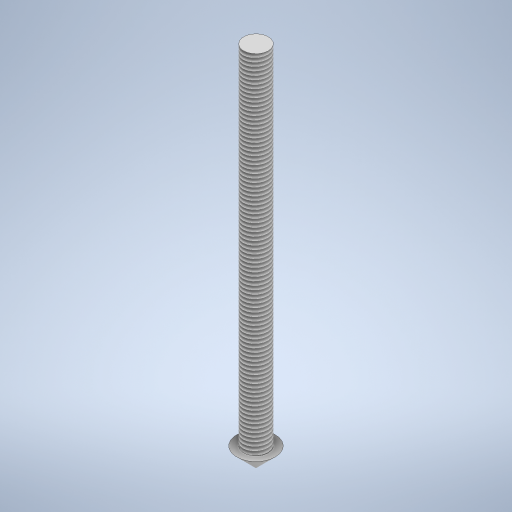
# Autodesk Inventor part: Digging Tool
Saved by Autodesk Inventor 2024 (Build 280153000, 153)
## iProperties
Created: 2024-02-05
Part Number: Digging Tool
Material: Generic
Document SubType Name: Modeling
Designer: Ramji Yadav
Density: 1 g/cm^3
Appearance: Default
Author: Ramji Yadav
Autodesk Inventor part; units mm, degrees
ref_plane "YZ Plane" through (0, 0, 0) normal (1, 0, 0) x (0, 1, 0)
ref_plane "XZ Plane" through (0, 0, 0) normal (0, 1, 0) x (-1, 0, 0)
ref_plane "XY Plane" through (0, 0, 0) normal (0, 0, 1) x (1, 0, 0)
sketch "Sketch1" plane through (0, 0, 0) normal (0, 0, 1) x (1, 0, 0)
  line L0 (0, 0) -> (10, 0)
  line L1 (0, 0) -> (0, -10)
  line L2 (0, -10) -> (10, 0)
  dimension "d0" = 10
  dimension "d1" = 10
  constraints: 6 end point, 1 horizontal, 1 vertical
  measures "d0" distance of L0.start L0.end
  measures "d1" distance of L0.start L1.end
revolve "Revolution1" add sketch "Sketch1" angle 360 about axis through (0, 0, 0) along (0, -1, 0)
sketch "Sketch2" plane through (0, 0, 0) normal (0, 1, 0) x (1, 0, 0)
  circle A0 centre (0, 0) radius 6.35
  dimension "d3" = 12.7
  constraints: 1 centre point, 1 coincident
  measures "d3" diameter of A0
extrude "Extrusion1" add sketch "Sketch2" along normal blind 180
thread "Thread1" size "M14x2" class "6g" standard "ANSI Metric M Profile" full length
body "Solid1"
